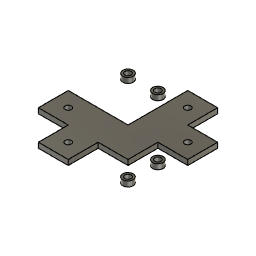
CampFireStoolInnerSully1 v1 (Autodesk Fusion 360 design; units mm, degrees)
Autodesk Fusion 360 part; units mm, degrees
sketch "Sketch1" plane through (0, 0, 0) normal (0, 0, 1) x (1, 0, 0)
  line L0 (146.05, -146.05) -> (-146.05, -146.05) construction
  line L1 (-146.05, -146.05) -> (-146.05, 146.05) construction
  line L2 (-146.05, 146.05) -> (146.05, 146.05) construction
  line L3 (146.05, 146.05) -> (146.05, -146.05) construction
  line L4 (146.05, -146.05) -> (-146.05, 146.05) construction
  line L5 (-146.05, -146.05) -> (146.05, 146.05) construction
  line L6 (0, -146.05) -> (0, 0) construction
  line L7 (0, 0) -> (0, 146.05) construction
  line L8 (0, 0) -> (-146.05, 0)
  line L9 (0, 0) -> (146.05, 0) construction
  line L10 (-73.025, 0) -> (-73.025, -146.05) construction
  line L11 (73.025, 0) -> (73.025, -146.05) construction
  line L12 (73.025, 0) -> (73.025, 146.05) construction
  line L13 (-73.025, 0) -> (-73.025, 146.05) construction
  line L14 (0, -73.025) -> (146.05, -73.025) construction
  line L15 (0, -73.025) -> (-146.05, -73.025) construction
  line L16 (0, 73.025) -> (-146.05, 73.025) construction
  line L17 (0, 73.025) -> (146.05, 73.025) construction
  line L18 (-146.05, 73.025) -> (-146.05, -73.025)
  line L19 (-146.05, -73.025) -> (-73.025, -73.025)
  line L20 (-73.025, -73.025) -> (-73.025, -146.05)
  line L21 (-73.025, -146.05) -> (0, -146.05)
  line L22 (0, -146.05) -> (0, -73.025)
  line L23 (0, -73.025) -> (73.025, -73.025)
  line L24 (73.025, -73.025) -> (73.025, 0)
  line L25 (73.025, 0) -> (146.05, 0)
  line L26 (146.05, 0) -> (146.05, 73.025)
  line L27 (146.05, 73.025) -> (73.025, 73.025)
  line L28 (73.025, 73.025) -> (73.025, 146.05)
  line L29 (73.025, 146.05) -> (0, 146.05)
  line L30 (0, 146.05) -> (0, 73.025)
  line L31 (0, 73.025) -> (0, 0)
  line L32 (0, 0) -> (-73.025, 0)
  line L33 (-73.025, 0) -> (-73.025, 73.025)
  line L34 (-73.025, 73.025) -> (-146.05, 73.025)
  line L35 (73.025, 109.5375) -> (0, 109.5375) construction
  line L36 (36.5125, 146.05) -> (36.5125, 109.5375) construction
  line L37 (109.5375, 73.025) -> (109.5375, 0) construction
  line L38 (146.05, 36.5125) -> (109.5375, 36.5125) construction
  line L39 (-73.025, -109.5375) -> (0, -109.5375) construction
  line L40 (-36.5125, -146.05) -> (-36.5125, -109.5375) construction
  line L41 (-109.5375, -73.025) -> (-109.5375, 0) construction
  line L42 (-146.05, -73.025) -> (-146.05, 0)
  line L43 (-146.05, -36.5125) -> (-109.5375, -36.5125) construction
  circle A0 centre (36.5125, 109.5375) radius 7.62
  circle A1 centre (109.5375, 36.5125) radius 7.62
  circle A2 centre (-109.5375, -36.5125) radius 7.62
  circle A3 centre (-36.5125, -109.5375) radius 7.62
  line L44 (0, 109.5375) -> (-146.05, 109.5375) construction
  line L45 (109.5375, 0) -> (109.5375, -146.05) construction
  line L46 (-73.025, 73.025) -> (0, 146.05) construction
  line L47 (73.025, -73.025) -> (146.05, 0) construction
  circle A4 centre (-36.5125, 109.5375) radius 12.7
  circle A5 centre (-109.5375, 109.5375) radius 12.7
  circle A6 centre (109.5375, -36.5125) radius 12.7
  circle A7 centre (109.5375, -109.5375) radius 12.7
  circle A8 centre (-109.5375, 109.5375) radius 7.62
  circle A9 centre (-36.5125, 109.5375) radius 7.62
  circle A10 centre (109.5375, -36.5125) radius 7.62
  circle A11 centre (109.5375, -109.5375) radius 7.62
  dimension "d1" = 292.1
  dimension "d2" = 292.1
  dimension "d3" = 15.24
  dimension "d4" = 15.24
  dimension "d5" = 15.24
  dimension "d6" = 15.24
  dimension "d7" = 25.4
  dimension "d8" = 25.4
  dimension "d9" = 25.4
  dimension "d10" = 25.4
  dimension "d11" = 15.24
  dimension "d12" = 15.24
  dimension "d13" = 15.24
  dimension "d14" = 15.24
  constraint horizontal L0
  constraint perpendicular L0 L1
  constraint parallel L0 L2
  constraint parallel L1 L3
  constraint coincident L4 L6.end
  constraint coincident L5 L6.end
  constraint coincident L6.end L7.start
  constraint midpoint L0 L6.start
  constraint midpoint L2 L7.end
  constraint midpoint L1 L8.end
  constraint midpoint L3 L9.end
  constraint midpoint L8 L10.start
  constraint coincident L0 L10.end
  constraint perpendicular L0 L10
  constraint midpoint L9 L11.start
  constraint coincident L0 L11.end
  constraint perpendicular L0 L11
  constraint coincident L2 L12.end
  constraint perpendicular L2 L12
  constraint coincident L2 L13.end
  constraint perpendicular L2 L13
  constraint midpoint L6 L14.start
  constraint coincident L3 L14.end
  constraint perpendicular L3 L14
  constraint coincident L1 L15.end
  constraint perpendicular L1 L15
  constraint midpoint L7 L16.start
  constraint coincident L1 L16.end
  constraint perpendicular L1 L16
  constraint coincident L3 L17.end
  constraint perpendicular L3 L17
  constraint midpoint L15 L19.end
  constraint midpoint L11 L23.end
  constraint midpoint L12 L27.end
  constraint midpoint L16 L33.end
  constraint midpoint L28 L35.start
  constraint midpoint L30 L35.end
  constraint midpoint L29 L36.start
  constraint midpoint L35 L36.end
  constraint midpoint L27 L37.start
  constraint midpoint L25 L37.end
  constraint midpoint L26 L38.start
  constraint midpoint L37 L38.end
  constraint midpoint L20 L39.start
  constraint midpoint L22 L39.end
  constraint midpoint L21 L40.start
  constraint midpoint L39 L40.end
  constraint midpoint L19 L41.start
  constraint coincident L8 L41.end
  constraint perpendicular L8 L41
  constraint midpoint L42 L43.start
  constraint midpoint L41 L43.end
  constraint coincident L36.end A0.centre
  constraint coincident L38.end A1.centre
  constraint coincident L43.end A2.centre
  constraint coincident L40.end A3.centre
  constraint coincident L1 L44.end
  constraint perpendicular L1 L44
  constraint coincident L0 L45.end
  constraint perpendicular L0 L45
  constraint midpoint L46 A4.centre
  constraint coincident L44 A5.centre
  constraint coincident L4 A5.centre
  constraint midpoint L47 A6.centre
  constraint coincident L45 A7.centre
  constraint coincident L4 A7.centre
  constraint concentric A5 A8
  constraint concentric A4 A9
  constraint concentric A6 A10
  constraint concentric A7 A11
  measures "d1" distance of L1.end L2.end
  measures "d2" distance of L0.end L1.end
  measures "d3" diameter of A0
  measures "d4" diameter of A1
  measures "d5" diameter of A2
  measures "d6" diameter of A3
  measures "d7" diameter of A4
  measures "d8" diameter of A5
  measures "d9" diameter of A6
  measures "d10" diameter of A7
  measures "d11" diameter of A8
  measures "d12" diameter of A9
  measures "d13" diameter of A10
  measures "d14" diameter of A11
extrude "Extrude1" add sketch "Sketch1" along normal blind 12.7 contours L8 L18 L19 L20 L21 L22 L23 L24 L25 L26 L27 L28 L29 L30 L31 L32 L42 | A4 | A5 | A6 | A7 makes body 1 at (-96.9006, 108.273, 8.4667) makes body 2 at (-23.8756, 108.273, 8.4667) makes body 3 at (122.1744, -37.777, 8.4667) makes body 4 at (-24.3417, -48.6833, 0) makes body 5 at (122.1744, -110.802, 8.4667)
